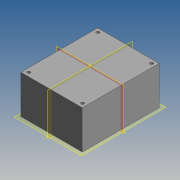
# Autodesk Inventor part: P028_PCB_surMesures
Saved by Autodesk Inventor 2021.3 (Build 253353000, 353)
## iProperties
Created: 2021-11-19
Part Number: P028_PCB_surMesures
Material: Générique
Document SubType Name: Modeling
Designer: gabri
Density: 1 g/cm^3
Appearance: Par défaut
Author: gabri
Autodesk Inventor part; units mm, degrees
sketch "Sketch2" plane through (0, 0, 0) normal (0, 0, 1) x (1, 0, 0)
  line L0 (40, -50) -> (-40, -50)
  line L1 (-40, -50) -> (-40, 50)
  line L2 (-40, 50) -> (40, 50)
  line L3 (40, 50) -> (40, -50)
  line L4 (40, -50) -> (-40, 50) construction
  line L5 (-40, -50) -> (40, 50) construction
  point P0 (0, 0)
  dimension "d0" = 100
  dimension "d1" = 80
  constraints: 12 end point, 2 midpoint, 2 parallel, 1 horizontal, 1 perpendicular
  measures "d0" distance of L0.end L1.end
  measures "d1" distance between parallel lines of L3 L1
extrude "Extrusion1" add sketch "Sketch2" along normal blind 50
sketch "Sketch3" plane through (0, 0, 50) normal (0, 0, 1) x (1, 0, 0)
  line L0 (40, 50) -> (-40, 50) construction
  line L1 (-40, 50) -> (-40, -50) construction
  line L2 (-40, -50) -> (40, -50) construction
  line L3 (40, -50) -> (40, 50) construction
  point P0 (0, 0)
  point P1 (-35, 45)
  point P2 (35, 45)
  point P3 (-35, -45)
  point P4 (35, -45)
  dimension "d4" = 5
  dimension "d5" = 5
  dimension "d6" = 5
  dimension "d7" = 5
  dimension "d8" = 5
  dimension "d9" = 5
  dimension "d10" = 5
  dimension "d11" = 5
  measures "d4" distance from line of L2 point (-35, -45)
  measures "d5" distance from line of L1 point (-35, -45)
  measures "d6" distance from line of L2 point (35, -45)
  measures "d7" distance from line of L3 point (35, -45)
  measures "d8" distance from line of L0 point (-35, 45)
  measures "d9" distance from line of point (-35, 45) L1
  measures "d10" distance from line of L0 point (35, 45)
  measures "d11" distance from line of L3 point (35, 45)
hole "Hole1" at (-35, 45, 50) at (35, 45, 50) at (-35, -45, 50) at (35, -45, 50) direction (0, 0, -1) diameter 4 depth 50
body "Solid1"
